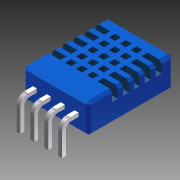
# Autodesk Inventor part: DHT11
Saved by Autodesk Inventor 2012 (Build 160160000, 160)
## iProperties
Created: 2015-01-21
Part Number: DHT11
Material: Default
Document SubType Name: Modeling
Designer: Anon
Density: 1 g/cm^3
Author: Anon
Autodesk Inventor part; units mm, degrees
ref_plane "YZ Plane" through (0, 0, 0) normal (1, 0, 0) x (0, 1, 0)
ref_plane "XZ Plane" through (0, 0, 0) normal (0, 1, 0) x (-1, 0, 0)
ref_plane "XY Plane" through (0, 0, 0) normal (0, 0, 1) x (1, 0, 0)
sketch "Sketch1" plane through (0, 0, 0) normal (0, 0, 1) x (1, 0, 0)
  line L0 (-6, 7.75) -> (6, 7.75)
  line L1 (6, 7.75) -> (6, -7.75)
  line L2 (6, -7.75) -> (-6, -7.75)
  line L3 (-6, -7.75) -> (-6, 7.75)
  point P0 (0, 0)
  dimension "d0" = 12
  dimension "d1" = 15.5
  dimension "d2" = 7.75
  dimension "d3" = 6
  constraints: 8 end point, 2 parallel, 1 horizontal, 1 perpendicular
  measures "d0" distance between parallel lines of L1 L3
  measures "d1" distance between parallel lines of L2 L0
  measures "d2" distance from line of point (0, 0) L2
  measures "d3" distance from line of point (0, 0) L3
extrude "Extrusion1" add sketch "Sketch1" along normal blind 5.5
sketch "Sketch2" plane through (0, 0, 5.5) normal (0, 0, 1) x (1, 0, 0)
  line L0 (-6, -7.75) -> (-6, 7.75) projected
  line L1 (-6, 5.6) -> (-3.4, 5.6)
  line L2 (-3.4, 5.6) -> (-3.4, 4.5)
  line L3 (-3.4, 4.5) -> (-6, 4.5)
  line L4 (-6, 4.5) -> (-6, 5.6)
  line L5 (-6, 3.6) -> (-3.4, 3.6)
  line L6 (-3.4, 3.6) -> (-3.4, 2.5)
  line L7 (-3.4, 2.5) -> (-6, 2.5)
  line L8 (-6, 2.5) -> (-6, 3.6)
  line L9 (-6, 1.6) -> (-3.4, 1.6)
  line L10 (-3.4, 1.6) -> (-3.4, 0.5)
  line L11 (-3.4, 0.5) -> (-6, 0.5)
  line L12 (-6, 0.5) -> (-6, 1.6)
  line L13 (-6, -0.4) -> (-3.4, -0.4)
  line L14 (-3.4, -0.4) -> (-3.4, -1.5)
  line L15 (-3.4, -1.5) -> (-6, -1.5)
  line L16 (-6, -1.5) -> (-6, -0.4)
  line L17 (-6, -2.4) -> (-3.4, -2.4)
  line L18 (-3.4, -2.4) -> (-3.4, -3.5)
  line L19 (-3.4, -3.5) -> (-6, -3.5)
  line L20 (-6, -3.5) -> (-6, -2.4)
  line L21 (0, 0) -> (0, 9.3585)
  line L22 (6, 5.6) -> (3.4, 5.6)
  line L23 (3.4, 5.6) -> (3.4, 4.5)
  line L24 (3.4, 4.5) -> (6, 4.5)
  line L25 (6, 4.5) -> (6, 5.6)
  line L26 (6, 3.6) -> (3.4, 3.6)
  line L27 (3.4, 3.6) -> (3.4, 2.5)
  line L28 (3.4, 2.5) -> (6, 2.5)
  line L29 (6, 2.5) -> (6, 3.6)
  line L30 (6, 1.6) -> (3.4, 1.6)
  line L31 (3.4, 1.6) -> (3.4, 0.5)
  line L32 (3.4, 0.5) -> (6, 0.5)
  line L33 (6, 0.5) -> (6, 1.6)
  line L34 (6, -0.4) -> (3.4, -0.4)
  line L35 (3.4, -0.4) -> (3.4, -1.5)
  line L36 (3.4, -1.5) -> (6, -1.5)
  line L37 (6, -1.5) -> (6, -0.4)
  line L38 (6, -2.4) -> (3.4, -2.4)
  line L39 (3.4, -2.4) -> (3.4, -3.5)
  line L40 (3.4, -3.5) -> (6, -3.5)
  line L41 (6, -3.5) -> (6, -2.4)
  line L42 (-2.525, 5.6) -> (-1.425, 5.6)
  line L43 (-1.425, 5.6) -> (-1.425, 4.5)
  line L44 (-1.425, 4.5) -> (-2.525, 4.5)
  line L45 (-2.525, 4.5) -> (-2.525, 5.6)
  line L46 (2.525, 5.6) -> (1.425, 5.6)
  line L47 (1.425, 5.6) -> (1.425, 4.5)
  line L48 (1.425, 4.5) -> (2.525, 4.5)
  line L49 (2.525, 4.5) -> (2.525, 5.6)
  line L50 (-0.55, 5.6) -> (0.55, 5.6)
  line L51 (0.55, 5.6) -> (0.55, 4.5)
  line L52 (0.55, 4.5) -> (-0.55, 4.5)
  line L53 (-0.55, 4.5) -> (-0.55, 5.6)
  line L54 (-2.525, 3.6) -> (-1.425, 3.6)
  line L55 (-1.425, 3.6) -> (-1.425, 2.5)
  line L56 (-1.425, 2.5) -> (-2.525, 2.5)
  line L57 (-2.525, 2.5) -> (-2.525, 3.6)
  line L58 (2.525, 3.6) -> (1.425, 3.6)
  line L59 (1.425, 3.6) -> (1.425, 2.5)
  line L60 (1.425, 2.5) -> (2.525, 2.5)
  line L61 (2.525, 2.5) -> (2.525, 3.6)
  line L62 (-0.55, 3.6) -> (0.55, 3.6)
  line L63 (0.55, 3.6) -> (0.55, 2.5)
  line L64 (0.55, 2.5) -> (-0.55, 2.5)
  line L65 (-0.55, 2.5) -> (-0.55, 3.6)
  line L66 (-2.525, 1.6) -> (-1.425, 1.6)
  line L67 (-1.425, 1.6) -> (-1.425, 0.5)
  line L68 (-1.425, 0.5) -> (-2.525, 0.5)
  line L69 (-2.525, 0.5) -> (-2.525, 1.6)
  line L70 (2.525, 1.6) -> (1.425, 1.6)
  line L71 (1.425, 1.6) -> (1.425, 0.5)
  line L72 (1.425, 0.5) -> (2.525, 0.5)
  line L73 (2.525, 0.5) -> (2.525, 1.6)
  line L74 (-0.55, 1.6) -> (0.55, 1.6)
  line L75 (0.55, 1.6) -> (0.55, 0.5)
  line L76 (0.55, 0.5) -> (-0.55, 0.5)
  line L77 (-0.55, 0.5) -> (-0.55, 1.6)
  line L78 (-2.525, -0.4) -> (-1.425, -0.4)
  line L79 (-1.425, -0.4) -> (-1.425, -1.5)
  line L80 (-1.425, -1.5) -> (-2.525, -1.5)
  line L81 (-2.525, -1.5) -> (-2.525, -0.4)
  line L82 (2.525, -0.4) -> (1.425, -0.4)
  line L83 (1.425, -0.4) -> (1.425, -1.5)
  line L84 (1.425, -1.5) -> (2.525, -1.5)
  line L85 (2.525, -1.5) -> (2.525, -0.4)
  line L86 (-0.55, -0.4) -> (0.55, -0.4)
  line L87 (0.55, -0.4) -> (0.55, -1.5)
  line L88 (0.55, -1.5) -> (-0.55, -1.5)
  line L89 (-0.55, -1.5) -> (-0.55, -0.4)
  line L90 (-2.525, -2.4) -> (-1.425, -2.4)
  line L91 (-1.425, -2.4) -> (-1.425, -3.5)
  line L92 (-1.425, -3.5) -> (-2.525, -3.5)
  line L93 (-2.525, -3.5) -> (-2.525, -2.4)
  line L94 (2.525, -2.4) -> (1.425, -2.4)
  line L95 (1.425, -2.4) -> (1.425, -3.5)
  line L96 (1.425, -3.5) -> (2.525, -3.5)
  line L97 (2.525, -3.5) -> (2.525, -2.4)
  line L98 (-0.55, -2.4) -> (0.55, -2.4)
  line L99 (0.55, -2.4) -> (0.55, -3.5)
  line L100 (0.55, -3.5) -> (-0.55, -3.5)
  line L101 (-0.55, -3.5) -> (-0.55, -2.4)
  dimension "d6" = 2.6
  dimension "d7" = 1.1
  dimension "d8" = 4.5
  dimension "d11" = 2
  dimension "d16" = 1.1
  dimension "d17" = 1.1
  dimension "d18" = 1.1
  dimension "d19" = 0.875
  dimension "d20" = 0.875
  dimension "d21" = 0.875
  dimension "d24" = 2
  constraints: 202 end point, 20 symmetric about line, 9 parallel, 4 horizontal, 4 perpendicular, 2 vertical, 1 point on line, 128 other
  measures "d6" distance of L2.end L3.end
  measures "d7" distance between parallel lines of L3 L1
  measures "d8" distance from line of L21.start L3
  measures "d11" distance of L1.start L5.start
  measures "d16" distance of L43.end L44.end
  measures "d17" distance of L48.end L47.end
  measures "d18" distance of L51.end L52.end
  measures "d19" distance between parallel lines of L2 L45
  measures "d20" distance between parallel lines of L53 L43
  measures "d21" distance between parallel lines of L47 L51
  measures "d24" distance of L44.end L56.end
extrude "Extrusion2" cut sketch "Sketch2" against normal blind 2
chamfer "Chamfer1" distance 0.5 angle 45 22 edges at (6, -1.95, 5.5) (6, -5.625, 5.5) (6, 0.05, 5.5) (6, 2.05, 5.5) (6, 4.05, 5.5) (6, 6.675, 5.5) (0, -7.75, 5.5) (0, 7.75, 5.5) (-6, 6.675, 5.5) (-6, 4.05, 5.5) (-6, 2.05, 5.5) (-6, 0.05, 5.5) (-6, -1.95, 5.5) (-6, -5.625, 5.5) (-6, 0, 0) (-6, -7.75, 2.75) (0, -7.75, 0) (6, -7.75, 2.75) (6, 0, 0) (-6, 7.75, 2.75) (6, 7.75, 2.75) (0, 7.75, 0)
sketch "Sketch3" plane through (0, 0, 0) normal (0, 0, -1) x (-1, 0, 0)
  line L0 (-2.3, 4.8) -> (-1.2, 4.8)
  line L1 (-1.2, 4.8) -> (-1.2, -3.2)
  line L2 (-1.2, -3.2) -> (-2.3, -3.2)
  line L3 (-2.3, -3.2) -> (-2.3, 4.8)
  line L4 (0, 0) -> (0, 8.5342) construction
  line L5 (2.3, 4.8) -> (1.2, 4.8)
  line L6 (1.2, 4.8) -> (1.2, -3.2)
  line L7 (1.2, -3.2) -> (2.3, -3.2)
  line L8 (2.3, -3.2) -> (2.3, 4.8)
  dimension "d34" = 1.1
  dimension "d35" = 8
  dimension "d36" = 1.2
  dimension "d37" = 4.8
  constraints: 18 end point, 4 symmetric about line, 3 parallel, 1 horizontal, 1 perpendicular
  measures "d34" distance of L1.end L2.end
  measures "d35" distance of L0.end L1.end
  measures "d36" distance from line of L4.start L1
  measures "d37" distance from line of L4.start L0
extrude "Extrusion3" cut sketch "Sketch3" against normal blind 2
sketch "Sketch4" plane through (-5.5, -7.75, 5) normal (0, -1, 0) x (1, 0, 0)
  line L0 (0, 0) -> (11, 0) projected
  line L1 (2.04, -2.6) -> (1.34, -2.6)
  line L2 (1.34, -2.6) -> (1.34, -1.9)
  line L3 (1.34, -1.9) -> (2.04, -1.9)
  line L4 (2.04, -1.9) -> (2.04, -2.6)
  line L5 (4.58, -2.6) -> (3.88, -2.6)
  line L6 (3.88, -2.6) -> (3.88, -1.9)
  line L7 (3.88, -1.9) -> (4.58, -1.9)
  line L8 (4.58, -1.9) -> (4.58, -2.6)
  line L9 (7.12, -2.6) -> (6.42, -2.6)
  line L10 (6.42, -2.6) -> (6.42, -1.9)
  line L11 (6.42, -1.9) -> (7.12, -1.9)
  line L12 (7.12, -1.9) -> (7.12, -2.6)
  line L13 (9.66, -2.6) -> (8.96, -2.6)
  line L14 (8.96, -2.6) -> (8.96, -1.9)
  line L15 (8.96, -1.9) -> (9.66, -1.9)
  line L16 (9.66, -1.9) -> (9.66, -2.6)
  point P0 (5.5, -5)
  dimension "d40" = 0.7
  dimension "d41" = 0.7
  dimension "d44" = 2.54
  dimension "d49" = 0.92
  dimension "d50" = 2.4
  constraints: 32 end point, 2 horizontal, 2 parallel, 1 perpendicular, 24 other
  measures "d40" distance between parallel lines of L4 L2
  measures "d41" distance between parallel lines of L1 L3
  measures "d44" distance of L1.start L5.start
  measures "d49" distance from line of point (5.5, -5) L8
  measures "d50" distance from line of point (5.5, -5) L5
extrude "Extrusion4" add sketch "Sketch4" along normal blind 8
sketch "Sketch5" plane through (-5.5, -15.75, 5) normal (0, -1, 0) x (1, 0, 0)
  line L0 (10.4469, -3.553) -> (0.6331, -3.553)
  line L1 (0.6331, -3.553) -> (0.6331, -0.9772)
  line L2 (0.6331, -0.9772) -> (10.4469, -0.9772)
  line L3 (10.4469, -0.9772) -> (10.4469, -3.553)
  point P0 (5.5, -5)
  constraints: 8 end point, 2 parallel, 1 horizontal, 1 perpendicular
extrude "Extrusion5" cut sketch "Sketch5" against normal blind 5
sketch "Sketch6" plane through (4.16, -7.75, 2.4) normal (0, 0, -1) x (-1, 0, 0)
  line L0 (0, -3) -> (0.7, -3) projected
  line L1 (0.7, 0) -> (0.7, -3) projected
  line L2 (0, -3) -> (0.7, -3)
  line L3 (0.7, -3) -> (0.7, -2.3)
  line L4 (0.7, -2.3) -> (0, -2.3)
  line L5 (0, -2.3) -> (0, -3)
  point P0 (4.16, 7.75)
  dimension "d55" = 0.7
  constraints: 8 end point, 2 parallel, 1 horizontal, 1 perpendicular, 1 point on line
  measures "d55" distance of L3.end L2.end
extrude "Extrusion6" add sketch "Sketch6" along normal blind 5
pattern_linear "Rectangular Pattern2" count 4 spacing 2.54 along (-1, 0, 0) of "Extrusion6"
fillet "Fillet3" radius 1.5 4 edges at (3.81, -10.75, 3.1) (-3.81, -10.75, 3.1) (-1.27, -10.75, 3.1) (1.27, -10.75, 3.1)
fillet "Fillet4" radius 0.9 4 edges at (-3.81, -10.05, 2.4) (-1.27, -10.05, 2.4) (1.27, -10.05, 2.4) (3.81, -10.05, 2.4)
body "Solid1"
